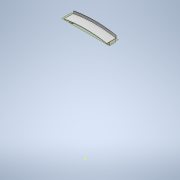
# Autodesk Inventor part: arc_de_cercle
Saved by Autodesk Inventor 2020.2 (Build 242310000, 310)
## iProperties
Created: 2020-01-28
Part Number: arc_de_cercle
Material: Générique
Document SubType Name: Modeling
Designer: anton
Density: 1 g/cm^3
Appearance: Par défaut
Author: anton
Autodesk Inventor part; units mm, degrees
ref_plane "YZ Plane" through (0, 0, 0) normal (1, 0, 0) x (0, 1, 0)
ref_plane "XZ Plane" through (0, 0, 0) normal (0, 1, 0) x (-1, 0, 0)
ref_plane "XY Plane" through (0, 0, 0) normal (0, 0, 1) x (1, 0, 0)
sketch "Esquisse1" plane through (0, 0, 0) normal (0, 0, 1) x (1, 0, 0)
  line L0 (-150.5839, 785.7) -> (150.5839, 785.7)
  arc A0 (150.5839, 785.7) -> (-150.5839, 785.7) centre (0, 0) ccw
  line L1 (-150.5839, 782.7) -> (150.5839, 782.7)
  line L2 (0, 797) -> (-150.5839, 797)
  arc A1 (150.5839, 782.7) -> (-150.5839, 782.7) centre (0, -3) ccw
  line L3 (-150.5839, 785.7) -> (-150.5839, 782.7)
  line L4 (150.5839, 785.7) -> (150.5839, 782.7)
  point P0 (0, 0)
  dimension "d4" = 785.7
  dimension "d8" = 3
  dimension "d9" = 14.3
  constraints: 10 end point, 5 point on circle, 3 horizontal, 2 centre point, 1 perpendicular
  measures "d4" distance from line of point (0, 0) L0
  measures "d8" distance between parallel lines of L0 L1
  measures "d9" distance between parallel lines of L1 L2
extrude "Extrusion1" add sketch "Esquisse1" along normal blind 65 contours A0 L2 A1 L0 | L0 A1 L3 | A0 L0 A1 L2 | L0 L4 A1
ref_plane "Plan de construction1" through (-150.5839, 782.7, 65) normal (0, -1, 0) x (0, 0, -1)
sketch "Esquisse4" plane through (-150.5839, 782.7, 65) normal (0, -1, 0) x (0, 0, -1)
  line L0 (65, 301.1678) -> (65, 0) projected
  line L1 (30, 8) -> (65, 8)
  line L2 (65, 8) -> (65, 28)
  line L3 (65, 28) -> (30, 28)
  line L4 (30, 28) -> (30, 8)
  line L5 (65, 0) -> (0, 0) projected
  line L6 (65, 273.1678) -> (30, 273.1678)
  line L7 (30, 273.1678) -> (30, 293.1678)
  line L8 (30, 293.1678) -> (65, 293.1678)
  line L9 (65, 293.1678) -> (65, 273.1678)
  line L10 (65, 301.1678) -> (0, 301.1678) projected
  point P0 (65, 150.5839)
  point P1 (65, 8)
  dimension "d13" = 20
  dimension "d14" = 35
  dimension "d15" = 8
  dimension "d16" = 35
  dimension "d17" = 8
  dimension "d18" = 20
  constraints: 16 end point, 4 parallel, 2 horizontal, 2 perpendicular, 2 point on line
  measures "d13" distance of L3.end L1.start
  measures "d14" distance of L2.end L3.end
  measures "d15" distance between parallel lines of L5 L1
  measures "d16" distance of L6.start L6.end
  measures "d17" distance between parallel lines of L10 L8
  measures "d18" distance of L6.end L7.end
extrude "Extrusion2" add sketch "Esquisse4" against normal up to surface
sketch "Esquisse5" plane through (-150.5839, 782.7, 65) normal (0, -1, 0) x (1, 0, 0)
  line L0 (0, -65) -> (8, -65) projected
  line L1 (28, -30) -> (28, -65) projected
  line L2 (8, -65) -> (28, -65)
  line L3 (28, -65) -> (28, -30)
  line L4 (28, -30) -> (8, -30)
  line L5 (8, -30) -> (8, -65)
  line L6 (273.1678, -30) -> (293.1678, -30) projected
  line L7 (293.1678, -30) -> (293.1678, -65) projected
  line L8 (273.1678, -30) -> (293.1678, -30)
  line L9 (293.1678, -30) -> (293.1678, -65)
  line L10 (293.1678, -65) -> (273.1678, -65)
  line L11 (273.1678, -65) -> (273.1678, -30)
  point P0 (150.5839, -65)
  constraints: 16 end point, 4 parallel, 2 horizontal, 2 perpendicular
extrude "Extrusion3" add sketch "Esquisse5" along normal blind 30
sketch "Esquisse9" plane through (0, 0, 65) normal (0, 0, 1) x (1, 0, 0)
  point P0 (0, 0)
sketch "Esquisse10" plane through (-150.5839, 782.7, 65) normal (0, -1, 0) x (0, 0, -1)
  line L0 (65, 301.1678) -> (0, 301.1678) projected
  line L1 (65, 301.1678) -> (68, 301.1678)
  line L2 (68, 301.1678) -> (68, 0)
  line L3 (68, 0) -> (65, 0)
  line L4 (65, 0) -> (65, 301.1678)
  point P0 (65, 150.5839)
  dimension "d81" = 3
  constraints: 8 end point, 2 parallel, 1 horizontal, 1 perpendicular
  measures "d81" distance of L2.end L3.end
extrude "Extrusion4" add sketch "Esquisse10" against normal blind 50
sketch "Esquisse11" plane through (-122.5839, 782.7, 0) normal (0, 0, 1) x (1, 0, 0)
  line L0 (-39.3889, 14.3) -> (313.6941, 14.3)
  line L1 (412.3411, 0) -> (-114.6772, 0) projected
  line L2 (273.1678, 0) -> (273.1678, 3) projected
  arc A0 (273.1678, 0) -> (-28, 0) centre (122.5839, -785.7) ccw
  line L3 (-28, 0) -> (273.1678, 0)
  point P0 (122.5839, -782.7)
  dimension "d84" = 14.3
  constraints: 4 end point, 2 horizontal, 2 point on circle, 1 centre point
  measures "d84" distance between parallel lines of L0 L1
extrude "Extrusion5" cut sketch "Esquisse11" against normal blind 10
sketch "Esquisse12" plane through (0, 0, 0) normal (0, 0, 1) x (1, 0, 0)
  line L0 (-152.2915, 801.4) -> (214.4689, 801.4)
  line L1 (288.3408, 782.7) -> (-228.7627, 782.7) projected
  line L2 (-154.8908, 815.7) -> (200.1728, 815.7)
  line L3 (150.5839, 785.7) -> (150.5839, 832.7) projected
  line L4 (-150.5839, 785.7) -> (-150.5839, 832.7) projected
  arc A0 (150.5839, 801.4) -> (-150.5839, 801.4) centre (0, 15.7) ccw
  line L5 (-150.5839, 801.4) -> (-150.5839, 832.7)
  line L6 (-150.5839, 832.7) -> (150.5839, 832.7) projected
  line L7 (150.5839, 832.7) -> (150.5839, 801.4)
  point P0 (0, 0)
  dimension "d87" = 18.7
  dimension "d88" = 14.3
  constraints: 8 end point, 4 point on line, 2 horizontal, 2 point on circle, 1 centre point, 1 collinear, 1 perpendicular, 1 tangent
  measures "d87" distance between parallel lines of L1 L0
  measures "d88" distance between parallel lines of L2 L0
extrude "Extrusion6" cut sketch "Esquisse12" against normal blind 10 contours L4 L2 A0 | A0 L2 L3 | L4 L6 L3 L2
sketch "Esquisse13" plane through (0, 0, 0) normal (0, 0, -1) x (-1, 0, 0)
  line L0 (142.5839, 784.1911) -> (142.5839, 752.7) projected
  line L1 (122.5839, 787.5525) -> (122.5839, 752.7) projected
  arc A0 (142.5839, 784.1911) -> (122.5839, 787.5525) centre (0, -3) ccw
  line L2 (142.5839, 784.1911) -> (142.5839, 752.7)
  line L3 (122.5839, 752.7) -> (142.5839, 752.7) projected
  line L4 (122.5839, 752.7) -> (122.5839, 787.5525)
  arc A1 (150.5839, 782.7) -> (-150.5839, 782.7) centre (0, -3) ccw projected
  arc A2 (-142.5839, 784.1911) -> (-122.5839, 787.5525) centre (0, -3) ccw
  line L5 (-122.5839, 787.5525) -> (-122.5839, 752.7) projected
  line L6 (-122.5839, 787.5525) -> (-122.5839, 752.7)
  line L7 (-142.5839, 752.7) -> (-122.5839, 752.7) projected
  line L8 (-122.5839, 752.7) -> (-142.5839, 752.7)
  line L9 (-142.5839, 784.1911) -> (-142.5839, 752.7) projected
  line L10 (-142.5839, 752.7) -> (-142.5839, 784.1911)
  arc A3 (-122.5839, 787.5525) -> (-142.5839, 784.1911) centre (0, -3) ccw
  point P0 (0, 0)
  constraints: 10 end point, 8 point on circle, 3 centre point, 2 perpendicular, 2 vertical, 1 collinear, 1 concentric
extrude "Extrusion7" add sketch "Esquisse13" along normal blind 3 contours L0 L3 L1 A0 | L5 L7 L9 A1
